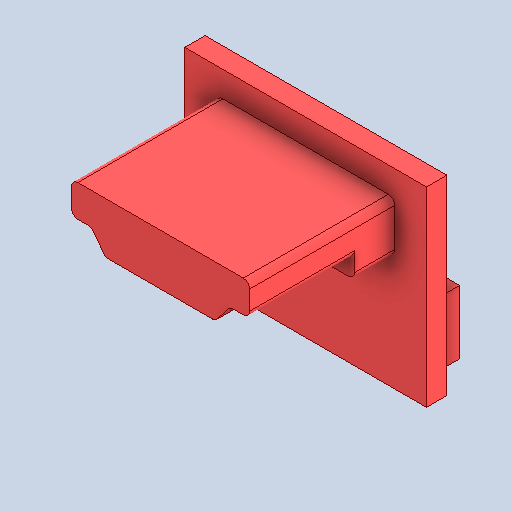
# Autodesk Inventor part: Adafruit_L_Bend_HDMI_Plug_Adapter_3550
Saved by Autodesk Inventor 2024.2 (Build 282272000, 272)
## iProperties
Created: 2020-06-16
Part Number: Adafruit_L_Bend_HDMI_Plug_Adapter_3550
Material: Generic
Document SubType Name: Modeling
Designer: Viktor Lindström
Density: 1 g/cm^3
Appearance: Default
Author: Viktor Lindström
Autodesk Inventor part; units mm, degrees
ref_plane "YZ Plane" through (0, 0, 0) normal (1, 0, 0) x (0, 1, 0)
ref_plane "XZ Plane" through (0, 0, 0) normal (0, 1, 0) x (-1, 0, 0)
sketch "Sketch1" plane through (0, 0, 0) normal (0, 0, 1) x (1, 0, 0)
  line L0 (-9.5, -7.5) -> (9.5, -7.5)
  line L1 (9.5, -7.5) -> (9.5, 7.5)
  line L2 (9.5, 7.5) -> (-9.5, 7.5)
  line L3 (-9.5, 7.5) -> (-9.5, -7.5)
  line L4 (-9.5, -7.5) -> (9.5, 7.5) construction
  line L5 (9.5, -7.5) -> (-9.5, 7.5) construction
  point P0 (0, 0)
  dimension "d0" = 19
  dimension "d1" = 15
  constraints: 12 end point, 2 midpoint, 2 parallel, 1 horizontal, 1 perpendicular
  measures "d0" distance between parallel lines of L1 L3
  measures "d1" distance between parallel lines of L2 L0
extrude "Extrusion1" add sketch "Sketch1" along normal blind 1.6
sketch "Sketch2" plane through (0, 0, 0) normal (0, 0, -1) x (-1, 0, 0)
  line L0 (0, -10.5) -> (0, 10.5) projected
  line L1 (-8.5, -6.5) -> (8.5, -6.5)
  line L2 (8.5, -6.5) -> (8.5, -1.5)
  line L3 (8.5, -1.5) -> (-8.5, -1.5)
  line L4 (-8.5, -1.5) -> (-8.5, -6.5)
  line L5 (-8.5, -6.5) -> (8.5, -1.5) construction
  line L6 (8.5, -6.5) -> (-8.5, -1.5) construction
  line L7 (9.5, -7.5) -> (-9.5, -7.5) projected
  point P0 (0, 0)
  point P1 (0, -4)
  dimension "d4" = 5
  dimension "d5" = 1
  dimension "d6" = 17
  constraints: 12 end point, 2 midpoint, 2 parallel, 1 horizontal, 1 perpendicular, 1 point on line
  measures "d4" distance between parallel lines of L3 L1
  measures "d5" distance between parallel lines of L7 L1
  measures "d6" distance between parallel lines of L2 L4
extrude "Extrusion2" add sketch "Sketch2" along normal blind 2
sketch "Sketch3" plane through (0, 0, 1.6) normal (0, 0, 1) x (1, 0, 0)
  line L0 (0, -10.5) -> (0, 10.5) projected
  line L1 (-7, 1.5) -> (7, 1.5)
  line L2 (7, 1.5) -> (7, 5.5)
  line L3 (7, 5.5) -> (-7, 5.5)
  line L4 (-7, 5.5) -> (-7, 1.5)
  line L5 (-7, 1.5) -> (7, 5.5) construction
  line L6 (7, 1.5) -> (-7, 5.5) construction
  line L7 (9.5, 7.5) -> (-9.5, 7.5) projected
  point P0 (0, 0)
  point P1 (0, 3.5)
  dimension "d9" = 14
  dimension "d10" = 4
  dimension "d11" = 2
  constraints: 12 end point, 2 midpoint, 2 parallel, 1 horizontal, 1 perpendicular, 1 point on line
  measures "d9" distance of L2.end L3.end
  measures "d10" distance between parallel lines of L1 L3
  measures "d11" distance between parallel lines of L7 L3
ref_plane "Work Plane1" through (0, 0, 13) normal (0, 0, -1) x (-1, 0, 0)
extrude "Extrusion3" add sketch "Sketch3" along normal up to surface (11.4 mm away)
sketch "Sketch4" plane through (-7, 1.5, 13) normal (0, 0, 1) x (1, 0, 0)
  line L0 (0, 4) -> (0, 0) projected
  line L1 (0, 0) -> (14, 0) projected
  line L2 (14, 0) -> (14, 4) projected
  line L3 (14, 4) -> (0, 4) projected
  line L4 (0, 1.492) -> (1.5696, 1.492)
  line L5 (1.5696, 1.492) -> (2.677, 0)
  line L6 (7, -12) -> (7, 9) construction
  line L7 (14, 1.492) -> (12.4304, 1.492)
  line L8 (12.4304, 1.492) -> (11.323, 0)
  point P0 (7, -1.5)
  constraints: 8 end point, 3 symmetric about line, 2 point on line, 1 horizontal
extrude "Extrusion4" cut sketch "Sketch4" against normal blind 8.25 contours L4 L5 L1 L0 | L2 L1 L8 L7
fillet "Fillet1" radius 0.5 10 edges at (7, 5.5, 7.3) (-7, 5.5, 7.3) (7, 2.992, 8.875) (4.323, 1.5, 8.875) (-7, 2.992, 8.875) (-4.323, 1.5, 8.875) (-5.4304, 2.992, 8.875) (5.4304, 2.992, 8.875) (7, 1.5, 3.175) (-7, 1.5, 3.175)
body "Solid1"
